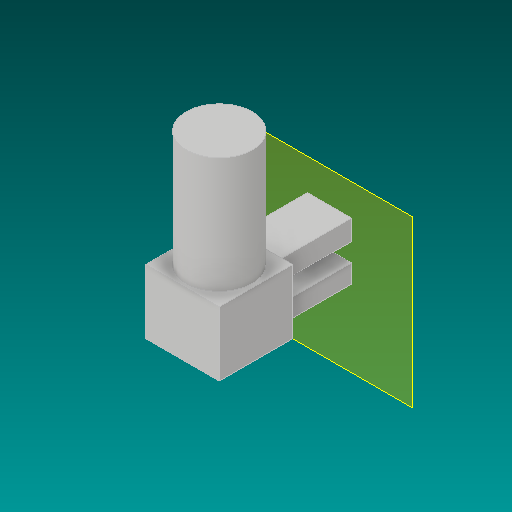
# Autodesk Inventor part: Joint_Wheel_Connect
Saved by Autodesk Inventor 2019 (Build 230136000, 136)
## iProperties
Created: 2020-12-14
Part Number: Joint_Wheel_Connect
Material: Generic
Document SubType Name: Modeling
Designer: Jason
Density: 1 g/cm^3
Appearance: Default
Mass: 4.49399 g
Surface Area: 21.6283 cm^2
Volume: 4.49399 cm^3
Author: Jason
Autodesk Inventor part; units mm, degrees
ref_plane "YZ Plane" through (0, 0, 0) normal (1, 0, 0) x (0, 1, 0)
ref_plane "XZ Plane" through (0, 0, 0) normal (0, 1, 0) x (-1, 0, 0)
ref_plane "XY Plane" through (0, 0, 0) normal (0, 0, 1) x (1, 0, 0)
ref_plane "Work Plane1" through (-10.8248, 8.3603, 0) normal (0, 0, 1) x (1, 0, 0)
sketch "Sketch1" plane through (-10.8248, 8.3603, 0) normal (0, 0, 1) x (1, 0, 0)
  line L0 (-3.81, 2.1338) -> (3.81, 2.1338) projected
  line L1 (3.81, 2.1338) -> (3.81, 5.3088) projected
  line L2 (3.81, 5.3088) -> (-3.81, 5.3088) projected
  line L3 (-3.81, 5.3088) -> (-3.81, 2.1338) projected
  line L4 (3.81, -1.0412) -> (-3.81, -1.0412) projected
  line L5 (-3.81, -1.0412) -> (-3.81, -4.2162) projected
  line L6 (-3.81, -4.2162) -> (3.81, -4.2162) projected
  line L7 (3.81, -4.2162) -> (3.81, -1.0412) projected
  line L8 (3.81, -1.0412) -> (-3.81, -1.0412)
  line L9 (-3.81, -1.0412) -> (-3.81, 2.1338)
  line L10 (-3.81, 2.1338) -> (3.81, 2.1338)
  line L11 (3.81, 2.1338) -> (3.81, -1.0412)
  line L12 (3.81, 5.3088) -> (-3.81, 5.3088)
  line L13 (-3.81, 5.3088) -> (-3.81, 8.8452)
  line L14 (-3.81, 8.8452) -> (3.81, 8.8452)
  line L15 (3.81, 8.8452) -> (3.81, 5.3088)
  point P0 (10.8248, -8.3603)
  constraints: 16 end point, 4 parallel, 2 horizontal, 2 perpendicular, 1 point on line
extrude "Extrusion1" add sketch "Sketch1" along normal blind 12.7 contours L0 L11 L4 L9 | L13 L14 L15 L2
sketch "Sketch2" plane through (-10.8248, 8.3603, 12.7) normal (0, 0, 1) x (1, 0, 0)
  line L0 (-6.35, -1.5875) -> (6.35, -1.5875)
  line L1 (6.35, -1.5875) -> (6.35, 9.525)
  line L2 (6.35, 9.525) -> (-6.35, 9.525)
  line L3 (-6.35, 9.525) -> (-6.35, -1.5875)
  point P0 (10.8248, -8.3603)
  constraints: 8 end point, 2 parallel, 1 horizontal, 1 perpendicular
extrude "Extrusion2" add sketch "Sketch2" along normal blind 12.7
sketch "Sketch4" plane through (-17.1748, 17.8853, 12.7) normal (0, -1, 0) x (1, 0, 0)
  circle A0 centre (6.35, 6.35) radius 5.715
  point P0 (17.1748, -12.7)
  dimension "d4" = 11.43
  constraints: 1 centre point
  measures "d4" diameter of A0
extrude "Extrusion3" add sketch "Sketch4" against normal blind 20
body "Solid1"
